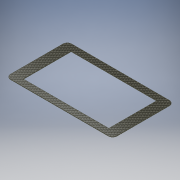
# Autodesk Inventor part: Display Lens
Saved by Autodesk Inventor 2017 SP1 (Build 210196100, 196)
## iProperties
Part Number: Display Lens
Material: Generisch
Document SubType Name: Modeling
Designer: u26048
Density: 1 g/cm^3
Appearance: Kohlenstofffaser 1
Author: u26048
Autodesk Inventor part; units mm, degrees
ref_plane "YZ Plane" through (0, 0, 0) normal (1, 0, 0) x (0, 1, 0)
ref_plane "XZ Plane" through (0, 0, 0) normal (0, 1, 0) x (-1, 0, 0)
ref_plane "XY Plane" through (0, 0, 0) normal (0, 0, 1) x (1, 0, 0)
sketch "Skizze1" plane through (0, 0, 0) normal (0, 0, 1) x (1, 0, 0)
  line L0 (-88.6, 55.38) -> (88.6, 55.38)
  line L1 (96.48, 47.5) -> (96.48, -47.5)
  line L2 (88.6, -55.38) -> (-88.6, -55.38)
  line L3 (-96.48, -47.5) -> (-96.48, 47.5)
  arc A0 (-88.6, 55.38) -> (-96.48, 47.5) centre (-88.6, 47.5) ccw
  arc A1 (-96.48, -47.5) -> (-88.6, -55.38) centre (-88.6, -47.5) ccw
  arc A2 (88.6, -55.38) -> (96.48, -47.5) centre (88.6, -47.5) ccw
  arc A3 (96.48, 47.5) -> (88.6, 55.38) centre (88.6, 47.5) ccw
  point P0 (0, 0)
  point P1 (96.48, -55.38)
  point P2 (96.48, 55.38)
  point P3 (-96.48, -55.38)
  point P4 (96.48, 0)
  point P5 (0, -55.38)
  dimension "d0" = 192.96
  dimension "d1" = 110.76
  dimension "d2" = 7.88
  constraints: 8 end point, 8 point on circle, 8 tangent, 6 point on line, 4 centre point, 3 equal radius, 2 midpoint, 2 parallel, 1 horizontal, 1 horizontal alignment, 1 perpendicular, 1 vertical alignment
  measures "d0" distance of point (96.48, -55.38) point (-96.48, -55.38)
  measures "d1" distance of point (96.48, 55.38) point (96.48, -55.38)
  measures "d2" radius of A0
extrude "Extrusion1" add sketch "Skizze1" against normal blind 0.7
sketch "Skizze2" plane through (0, 0, 0) normal (0, 0, 1) x (1, 0, 0)
  line L0 (-77.44, 43.36) -> (77.44, 43.36)
  line L1 (77.44, 43.36) -> (77.44, -43.36)
  line L2 (77.44, -43.36) -> (-77.44, -43.36)
  line L3 (-77.44, -43.36) -> (-77.44, 43.36)
  point P0 (0, 0)
  point P1 (77.44, 0)
  point P2 (0, 43.36)
  dimension "d5" = 154.88
  dimension "d6" = 86.72
  constraints: 8 end point, 2 midpoint, 2 parallel, 1 horizontal, 1 horizontal alignment, 1 perpendicular, 1 vertical alignment
  measures "d5" distance between parallel lines of L1 L3
  measures "d6" distance between parallel lines of L2 L0
extrude "Extrusion2" cut sketch "Skizze2" against normal up to surface (0.7 mm away)
